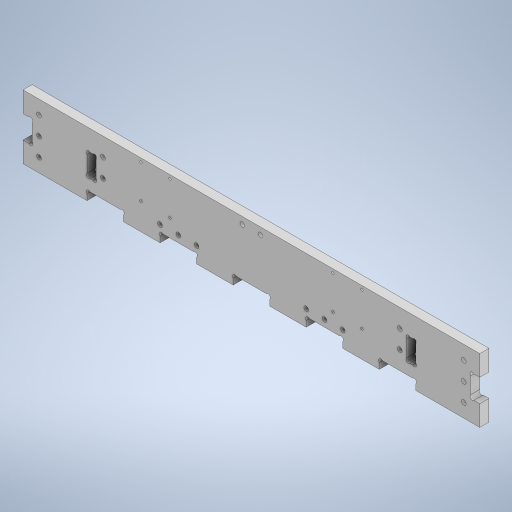
# Autodesk Inventor part: Back Wall
Saved by Autodesk Inventor 2023 (Build 270158000, 158)
## iProperties
Created: 2022-12-26
Part Number: Back Wall
Material: Generic
Document SubType Name: Modeling
Designer: justi
Density: 1 g/cm^3
Appearance: Default
Mass: 647.44 g
Surface Area: 1291.94 cm^2
Volume: 647.44 cm^3
Author: justi
Autodesk Inventor part; units mm, degrees
ref_plane "YZ Plane" through (0, 0, 0) normal (1, 0, 0) x (0, 1, 0)
ref_plane "XZ Plane" through (0, 0, 0) normal (0, 1, 0) x (-1, 0, 0)
ref_plane "XY Plane" through (0, 0, 0) normal (0, 0, 1) x (1, 0, 0)
sketch "Sketch1" plane through (0, 0, 0) normal (0, 0, 1) x (1, 0, 0)
  line L0 (0, 0) -> (457.2, 0)
  line L1 (457.2, 0) -> (457.2, 88.9)
  line L2 (457.2, 88.9) -> (0, 88.9)
  line L3 (0, 88.9) -> (0, 0)
  line L4 (0, 0) -> (50.8, 0)
  line L5 (50.8, 0) -> (50.8, 12.7)
  line L6 (50.8, 12.7) -> (0, 12.7)
  line L7 (0, 12.7) -> (0, 0)
  line L8 (457.2, 0) -> (406.4, 0)
  line L9 (406.4, 0) -> (406.4, 12.7)
  line L10 (406.4, 12.7) -> (457.2, 12.7)
  line L11 (457.2, 12.7) -> (457.2, 0)
  line L12 (101.6, 0) -> (152.4, 0)
  line L13 (152.4, 0) -> (152.4, 12.7)
  line L14 (152.4, 12.7) -> (101.6, 12.7)
  line L15 (101.6, 12.7) -> (101.6, 0)
  line L16 (355.6, 0) -> (304.8, 0)
  line L17 (304.8, 0) -> (304.8, 12.7)
  line L18 (304.8, 12.7) -> (355.6, 12.7)
  line L19 (355.6, 12.7) -> (355.6, 0)
  line L20 (254, 0) -> (203.2, 0)
  line L21 (203.2, 0) -> (203.2, 12.7)
  line L22 (203.2, 12.7) -> (254, 12.7)
  line L23 (254, 12.7) -> (254, 0)
  line L24 (0, 60.325) -> (12.7, 60.325)
  line L25 (12.7, 60.325) -> (12.7, 28.575)
  line L26 (12.7, 28.575) -> (0, 28.575)
  line L27 (0, 28.575) -> (0, 60.325)
  line L28 (457.2, 60.325) -> (444.5, 60.325)
  line L29 (444.5, 60.325) -> (444.5, 28.575)
  line L30 (444.5, 28.575) -> (457.2, 28.575)
  line L31 (457.2, 28.575) -> (457.2, 60.325)
  line L32 (0, 88.9) -> (-88.9, 88.9)
  line L33 (-88.9, 88.9) -> (-88.9, 0)
  line L34 (-88.9, 0) -> (0, 0)
  line L35 (0, 0) -> (0, 88.9)
  line L36 (-88.9, 60.325) -> (-76.2, 60.325)
  line L37 (-76.2, 60.325) -> (-76.2, 28.575)
  line L38 (-76.2, 28.575) -> (-88.9, 28.575)
  line L39 (-88.9, 28.575) -> (-88.9, 60.325)
  line L40 (457.2, 88.9) -> (546.1, 88.9)
  line L41 (546.1, 88.9) -> (546.1, 0)
  line L42 (546.1, 0) -> (457.2, 0)
  line L43 (457.2, 0) -> (457.2, 88.9)
  line L44 (546.1, 60.325) -> (533.4, 60.325)
  line L45 (533.4, 60.325) -> (533.4, 28.575)
  line L46 (533.4, 28.575) -> (546.1, 28.575)
  line L47 (546.1, 28.575) -> (546.1, 60.325)
  point P0 (0, 28.575)
  dimension "d0" = 457.2
  dimension "d1" = 88.9
  dimension "d2" = 50.8
  dimension "d3" = 12.7
  dimension "d4" = 50.8
  dimension "d5" = 12.7
  dimension "d6" = 50.8
  dimension "d7" = 12.7
  dimension "d8" = 50.8
  dimension "d9" = 50.8
  dimension "d10" = 12.7
  dimension "d11" = 50.8
  dimension "d12" = 50.8
  dimension "d13" = 12.7
  dimension "d14" = 50.8
  dimension "d15" = 12.7
  dimension "d16" = 15.875
  dimension "d17" = 28.575
  dimension "d18" = 12.7
  dimension "d19" = 28.575
  dimension "d20" = 15.875
  dimension "d21" = 88.9
  dimension "d22" = 12.7
  dimension "d23" = 28.575
  dimension "d24" = 31.75
  dimension "d25" = 88.9
  dimension "d26" = 12.7
  dimension "d27" = 28.575
  dimension "d28" = 31.75
  constraints: 96 end point, 24 parallel, 12 horizontal, 12 perpendicular, 7 point on line
  measures "d0" distance of L1.end L2.end
  measures "d1" distance of L0.end L1.end
  measures "d2" distance of L6.end L5.end
  measures "d3" distance of L4.end L5.end
  measures "d4" distance of L9.end L10.end
  measures "d5" distance of L8.end L9.end
  measures "d6" distance of L14.end L13.end
  measures "d7" distance of L12.end L13.end
  measures "d8" distance between parallel lines of L5 L15
  measures "d9" distance of L17.end L18.end
  measures "d10" distance of L16.end L17.end
  measures "d11" distance between parallel lines of L9 L19
  measures "d12" distance of L21.end L22.end
  measures "d13" distance of L20.end L21.end
  measures "d14" distance between parallel lines of L17 L23
  measures "d15" distance of L25.end L26.end
  measures "d16" distance between parallel lines of L6 L26
  measures "d17" distance between parallel lines of L2 L24
  measures "d18" distance of L30.end L29.end
  measures "d19" distance between parallel lines of L2 L28
  measures "d20" distance between parallel lines of L10 L30
  measures "d21" distance of L34.end L33.end
  measures "d22" distance of L37.end L38.end
  measures "d23" distance between parallel lines of L32 L36
  measures "d24" distance of L36.end L37.end
  measures "d25" distance of L41.end L42.end
  measures "d26" distance of L46.end L45.end
  measures "d27" distance between parallel lines of L40 L44
  measures "d28" distance of L44.end L45.end
extrude "Extrusion1" add sketch "Sketch1" along normal blind 12.7 contours L34 L33 L38 L37 L36 L32 L3 | L5 L6 L3 L26 L25 L24 L2 L1 L28 L29 L30 L10 L9 L0 L19 L18 L17 L23 L22 L21 L13 L14 L15 | L40 L41 L44 L45 L46 L42 L1
sketch "Sketch2" plane through (0, 0, 12.7) normal (0, 0, 1) x (1, 0, 0)
  line L0 (-76.2, 60.325) -> (-76.2, 28.575) projected
  line L1 (-76.2, 60.325) -> (-78.4451, 58.0799)
  line L2 (-76.2, 28.575) -> (-78.4451, 30.8201)
  line L3 (0, 28.575) -> (0, 60.325) projected
  line L4 (0, 60.325) -> (2.2451, 58.0799)
  line L5 (0, 60.325) -> (12.7, 60.325) projected
  line L6 (12.7, 60.325) -> (10.4549, 58.0799)
  line L7 (12.7, 60.325) -> (12.7, 28.575) projected
  line L8 (12.7, 28.575) -> (0, 28.575) projected
  line L9 (0, 28.575) -> (2.2451, 30.8201)
  line L10 (12.7, 60.325) -> (12.7, 28.575) projected
  line L11 (12.7, 28.575) -> (10.4549, 30.8201)
  line L12 (0, 0) -> (0, 12.7) projected
  line L13 (0, 12.7) -> (2.2451, 10.4549)
  line L14 (0, 12.7) -> (50.8, 12.7) projected
  line L15 (50.8, 12.7) -> (50.8, 0) projected
  line L16 (50.8, 12.7) -> (48.5549, 10.4549)
  line L17 (101.6, 0) -> (101.6, 12.7) projected
  line L18 (101.6, 12.7) -> (103.8451, 10.4549)
  line L19 (101.6, 12.7) -> (152.4, 12.7) projected
  line L20 (152.4, 12.7) -> (152.4, 0) projected
  line L21 (152.4, 12.7) -> (150.1549, 10.4549)
  line L22 (203.2, 0) -> (203.2, 12.7) projected
  line L23 (203.2, 12.7) -> (205.4451, 10.4549)
  line L24 (203.2, 12.7) -> (254, 12.7) projected
  line L25 (254, 12.7) -> (254, 0) projected
  line L26 (254, 12.7) -> (251.7549, 10.4549)
  line L27 (304.8, 0) -> (304.8, 12.7) projected
  line L28 (304.8, 12.7) -> (307.0451, 10.4549)
  line L29 (304.8, 12.7) -> (355.6, 12.7) projected
  line L30 (355.6, 12.7) -> (355.6, 0) projected
  line L31 (355.6, 12.7) -> (353.3549, 10.4549)
  line L32 (406.4, 0) -> (406.4, 12.7) projected
  line L33 (406.4, 12.7) -> (408.6451, 10.4549)
  line L34 (406.4, 12.7) -> (457.2, 12.7) projected
  line L35 (457.2, 12.7) -> (454.9549, 10.4549)
  line L36 (457.2, 12.7) -> (457.2, 0) projected
  line L37 (444.5, 28.575) -> (444.5, 60.325) projected
  line L38 (444.5, 60.325) -> (446.7451, 58.0799)
  line L39 (444.5, 60.325) -> (457.2, 60.325) projected
  line L40 (457.2, 60.325) -> (457.2, 28.575) projected
  line L41 (457.2, 60.325) -> (454.9549, 58.0799)
  line L42 (444.5, 28.575) -> (446.7451, 30.8201)
  line L43 (457.2, 28.575) -> (444.5, 28.575) projected
  line L44 (457.2, 28.575) -> (454.9549, 30.8201)
  line L45 (533.4, 28.575) -> (533.4, 60.325) projected
  line L46 (533.4, 60.325) -> (535.6451, 58.0799)
  line L47 (533.4, 60.325) -> (546.1, 60.325) projected
  line L48 (546.1, 28.575) -> (533.4, 28.575) projected
  line L49 (533.4, 28.575) -> (535.6451, 30.8201)
  circle A0 centre (-78.4451, 58.0799) radius 3.175
  circle A1 centre (-78.4451, 30.8201) radius 3.175
  circle A2 centre (2.2451, 58.0799) radius 3.175
  circle A3 centre (10.4549, 58.0799) radius 3.175
  circle A4 centre (2.2451, 30.8201) radius 3.175
  circle A5 centre (10.4549, 30.8201) radius 3.175
  circle A6 centre (2.2451, 10.4549) radius 3.175
  circle A7 centre (48.5549, 10.4549) radius 3.175
  circle A8 centre (103.8451, 10.4549) radius 3.175
  circle A9 centre (150.1549, 10.4549) radius 3.175
  circle A10 centre (205.4451, 10.4549) radius 3.175
  circle A11 centre (251.7549, 10.4549) radius 3.175
  circle A12 centre (307.0451, 10.4549) radius 3.175
  circle A13 centre (353.3549, 10.4549) radius 3.175
  circle A14 centre (408.6451, 10.4549) radius 3.175
  circle A15 centre (454.9549, 10.4549) radius 3.175
  circle A16 centre (446.7451, 30.8201) radius 3.175
  circle A17 centre (454.9549, 30.8201) radius 3.175
  circle A18 centre (454.9549, 58.0799) radius 3.175
  circle A19 centre (446.7451, 58.0799) radius 3.175
  circle A20 centre (535.6451, 58.0799) radius 3.175
  circle A21 centre (535.6451, 30.8201) radius 3.175
  dimension "d31" = 3.175
  dimension "d32" = 45
  dimension "d33" = 3.175
  dimension "d34" = 45
  dimension "d35" = 3.175
  dimension "d36" = 45
  dimension "d37" = 3.175
  dimension "d38" = 45
  dimension "d39" = 3.175
  dimension "d40" = 45
  dimension "d41" = 3.175
  dimension "d42" = 45
  dimension "d43" = 3.175
  dimension "d44" = 45
  dimension "d45" = 3.175
  dimension "d46" = 45
  dimension "d47" = 3.175
  dimension "d48" = 45
  dimension "d49" = 3.175
  dimension "d50" = 45
  dimension "d51" = 3.175
  dimension "d52" = 45
  dimension "d53" = 3.175
  dimension "d54" = 45
  dimension "d55" = 3.175
  dimension "d56" = 45
  dimension "d57" = 3.175
  dimension "d58" = 45
  dimension "d59" = 3.175
  dimension "d60" = 45
  dimension "d61" = 3.175
  dimension "d62" = 45
  dimension "d63" = 3.175
  dimension "d64" = 45
  dimension "d65" = 3.175
  dimension "d66" = 45
  dimension "d67" = 3.175
  dimension "d68" = 45
  dimension "d69" = 3.175
  dimension "d70" = 45
  dimension "d71" = 3.175
  dimension "d72" = 45
  dimension "d73" = 3.175
  dimension "d74" = 45
  dimension "d75" = 6.35
  dimension "d76" = 6.35
  dimension "d77" = 6.35
  dimension "d78" = 6.35
  dimension "d79" = 6.35
  dimension "d80" = 6.35
  dimension "d81" = 6.35
  dimension "d82" = 6.35
  dimension "d83" = 6.35
  dimension "d84" = 6.35
  dimension "d85" = 6.35
  dimension "d86" = 6.35
  dimension "d87" = 6.35
  dimension "d88" = 6.35
  dimension "d89" = 6.35
  dimension "d90" = 6.35
  dimension "d91" = 6.35
  dimension "d92" = 6.35
  dimension "d93" = 6.35
  dimension "d94" = 6.35
  constraints: 44 end point, 22 centre point, 14 point on line, 1 coincident
  measures "d31" distance of L0.start L1.end
  measures "d32" angle of L0 L1
  measures "d33" distance of L0.end L2.end
  measures "d34" angle of L0 L2
  measures "d35" distance of L3.end L4.end
  measures "d36" angle of L5 L4
  measures "d37" distance of L5.end L6.end
  measures "d38" angle of L7 L6
  measures "d39" distance of L3.start L9.end
  measures "d40" angle of L8 L9
  measures "d41" distance of L7.end L11.end
  measures "d42" angle of L7 L11
  measures "d43" distance of L12.end L13.end
  measures "d44" angle of L14 L13
  measures "d45" distance of L14.end L16.end
  measures "d46" angle of L15 L16
  measures "d47" distance of L17.end L18.end
  measures "d48" angle of L19 L18
  measures "d49" distance of L19.end L21.end
  measures "d50" angle of L20 L21
  measures "d51" distance of L22.end L23.end
  measures "d52" angle of L24 L23
  measures "d53" distance of L24.end L26.end
  measures "d54" angle of L25 L26
  measures "d55" distance of L27.end L28.end
  measures "d56" angle of L29 L28
  measures "d57" distance of L29.end L31.end
  measures "d58" angle of L30 L31
  measures "d59" distance of L32.end L33.end
  measures "d60" angle of L34 L33
  measures "d61" distance of L34.end L35.end
  measures "d62" angle of L36 L35
  measures "d63" distance of L37.end L38.end
  measures "d64" angle of L39 L38
  measures "d65" distance of L39.end L41.end
  measures "d66" angle of L40 L41
  measures "d67" distance of L37.start L42.end
  measures "d68" angle of L43 L42
  measures "d69" distance of L40.end L44.end
  measures "d70" angle of L40 L44
  measures "d71" distance of L45.end L46.end
  measures "d72" angle of L47 L46
  measures "d73" distance of L45.start L49.end
  measures "d74" angle of L48 L49
  measures "d75" diameter of A0
  measures "d76" diameter of A1
  measures "d77" diameter of A2
  measures "d78" diameter of A3
  measures "d79" diameter of A4
  measures "d80" diameter of A5
  measures "d81" diameter of A6
  measures "d82" diameter of A7
  measures "d83" diameter of A8
  measures "d84" diameter of A9
  measures "d85" diameter of A10
  measures "d86" diameter of A11
  measures "d87" diameter of A12
  measures "d88" diameter of A13
  measures "d89" diameter of A14
  measures "d90" diameter of A15
  measures "d91" diameter of A16
  measures "d92" diameter of A17
  measures "d93" diameter of A18
  measures "d94" diameter of A19
extrude "Extrusion2" cut sketch "Sketch2" against normal blind 12.7 contours A0 L0 | A1 L0 | L0 A1 | L0 A0 | A4 L3 | L3 A4 L8 | L8 A4 | A2 L3 | L3 L5 A2 | A5 L7 L8 | L8 A5 | A2 L5 | L7 A5 | A3 L5 L7 | L7 A3 | A3 L5 | A6 L12 | A7 L14 | L14 L15 A7 | L12 L14 A6 | A6 L14 | A7 L15 | A8 L17 | A9 L19 | L19 L20 A9 | L17 L19 A8 | A8 L19 | A9 L20 | A10 L22 | A11 L24 | L24 L25 A11 | L22 L24 A10 | A10 L24 | A11 L25 | A12 L27 | A13 L29 | L29 L30 A13 | L27 L29 A12 | A12 L29 | A13 L30 | A14 L32 | A15 L34 | L34 L36 A15 | L32 L34 A14 | A14 L34 | A15 L36 | A16 L37 | L37 A16 L43 | L43 A16 | A19 L37 | L37 L39 A19 | A17 L40 L43 | L43 A17 | A19 L39 | L40 A17 | A18 L39 L40 | L40 A18 | A18 L39 | A21 L45 | L45 A21 L48 | A20 L45 | L45 L47 A20 | L48 A21 | A20 L47
sketch "Sketch3" plane through (0, 0, 12.7) normal (0, 0, 1) x (1, 0, 0)
  circle A0 centre (127, 22.225) radius 3.175
  line L0 (106.0901, 12.7) -> (147.9099, 12.7) projected
  line L1 (101.6, 0) -> (101.6, 8.2099) projected
  circle A1 centre (101.6, 22.225) radius 3.175
  circle A2 centre (152.4, 22.225) radius 3.175
  circle A3 centre (330.2, 22.225) radius 3.175
  line L2 (309.2901, 12.7) -> (351.1099, 12.7) projected
  line L3 (355.6, 8.2099) -> (355.6, 0) projected
  circle A4 centre (304.8, 22.225) radius 3.175
  circle A5 centre (355.6, 22.225) radius 3.175
  circle A6 centre (22.225, 38.1) radius 3.175
  line L4 (4.4901, 12.7) -> (46.3099, 12.7) projected
  line L5 (12.7, 55.8349) -> (12.7, 33.0651) projected
  circle A7 centre (22.225, 63.5) radius 3.175
  circle A8 centre (434.975, 38.1) radius 3.175
  line L6 (444.5, 33.0651) -> (444.5, 55.8349) projected
  line L7 (410.8901, 12.7) -> (452.7099, 12.7) projected
  circle A9 centre (434.975, 63.5) radius 3.175
  circle A10 centre (-66.675, 44.45) radius 3.175
  line L8 (546.1, 88.9) -> (-88.9, 88.9) projected
  line L9 (-76.2, 55.8349) -> (-76.2, 33.0651) projected
  circle A11 centre (-66.675, 69.85) radius 3.175
  circle A12 centre (-66.675, 19.05) radius 3.175
  circle A13 centre (523.875, 44.45) radius 3.175
  line L10 (533.4, 33.0651) -> (533.4, 55.8349) projected
  circle A14 centre (523.875, 69.85) radius 3.175
  circle A15 centre (523.875, 19.05) radius 3.175
  point P0 (0, 0)
  dimension "d99" = 6.35
  dimension "d100" = 9.525
  dimension "d101" = 25.4
  dimension "d102" = 6.35
  dimension "d103" = 9.525
  dimension "d104" = 25.4
  dimension "d105" = 6.35
  dimension "d106" = 25.4
  dimension "d107" = 9.525
  dimension "d108" = 6.35
  dimension "d109" = 9.525
  dimension "d110" = 25.4
  dimension "d111" = 6.35
  dimension "d112" = 9.525
  dimension "d113" = 25.4
  dimension "d114" = 6.35
  dimension "d115" = 25.4
  dimension "d116" = 9.525
  dimension "d117" = 6.35
  dimension "d118" = 25.4
  dimension "d119" = 9.525
  dimension "d120" = 6.35
  dimension "d121" = 9.525
  dimension "d122" = 25.4
  dimension "d123" = 6.35
  dimension "d124" = 9.525
  dimension "d125" = 25.4
  dimension "d126" = 6.35
  dimension "d127" = 9.525
  dimension "d128" = 25.4
  dimension "d129" = 6.35
  dimension "d130" = 44.45
  dimension "d131" = 9.525
  dimension "d132" = 6.35
  dimension "d133" = 9.525
  dimension "d134" = 25.4
  dimension "d135" = 6.35
  dimension "d136" = 9.525
  dimension "d137" = 25.4
  dimension "d138" = 6.35
  dimension "d139" = 9.525
  dimension "d140" = 44.45
  dimension "d141" = 6.35
  dimension "d142" = 9.525
  dimension "d143" = 25.4
  dimension "d144" = 6.35
  dimension "d145" = 9.525
  dimension "d146" = 25.4
  constraints: 16 centre point
  measures "d99" diameter of A0
  measures "d100" distance from line of L0 A0.centre
  measures "d101" distance from line of L1 A0.centre
  measures "d102" diameter of A1
  measures "d103" distance from line of L0 A1.centre
  measures "d104" distance of A0.centre A1.centre
  measures "d105" diameter of A2
  measures "d106" distance of A0.centre A2.centre
  measures "d107" distance from line of L0 A2.centre
  measures "d108" diameter of A3
  measures "d109" distance from line of L2 A3.centre
  measures "d110" distance from line of L3 A3.centre
  measures "d111" diameter of A4
  measures "d112" distance from line of L2 A4.centre
  measures "d113" distance of A3.centre A4.centre
  measures "d114" diameter of A5
  measures "d115" distance of A3.centre A5.centre
  measures "d116" distance from line of L2 A5.centre
  measures "d117" diameter of A6
  measures "d118" distance from line of L4 A6.centre
  measures "d119" distance from line of L5 A6.centre
  measures "d120" diameter of A7
  measures "d121" distance from line of L5 A7.centre
  measures "d122" distance of A6.centre A7.centre
  measures "d123" diameter of A8
  measures "d124" distance from line of L6 A8.centre
  measures "d125" distance from line of L7 A8.centre
  measures "d126" diameter of A9
  measures "d127" distance from line of L6 A9.centre
  measures "d128" distance of A8.centre A9.centre
  measures "d129" diameter of A10
  measures "d130" distance from line of L8 A10.centre
  measures "d131" distance from line of L9 A10.centre
  measures "d132" diameter of A11
  measures "d133" distance from line of L9 A11.centre
  measures "d134" distance of A10.centre A11.centre
  measures "d135" diameter of A12
  measures "d136" distance from line of L9 A12.centre
  measures "d137" distance of A10.centre A12.centre
  measures "d138" diameter of A13
  measures "d139" distance from line of L10 A13.centre
  measures "d140" distance from line of L8 A13.centre
  measures "d141" diameter of A14
  measures "d142" distance from line of L10 A14.centre
  measures "d143" distance of A13.centre A14.centre
  measures "d144" diameter of A15
  measures "d145" distance from line of L10 A15.centre
  measures "d146" distance of A13.centre A15.centre
extrude "Extrusion3" cut sketch "Sketch3" against normal blind 12.7
sketch "Sketch6" plane through (0, 0, 12.7) normal (0, 0, 1) x (1, 0, 0)
  circle A0 centre (115.2922, 36.9094) radius 1.5875
  circle A1 centre (127, 22.225) radius 3.175 projected
  circle A2 centre (115.2922, 83.7406) radius 1.5875
  line L0 (88.9, 31.75) -> (165.1, 31.75)
  line L1 (165.1, 31.75) -> (165.1, 12.7)
  line L2 (165.1, 12.7) -> (88.9, 12.7)
  line L3 (88.9, 12.7) -> (88.9, 31.75)
  line L4 (88.9, 31.75) -> (165.1, 12.7) construction
  line L5 (165.1, 31.75) -> (88.9, 12.7) construction
  line L6 (546.1, 88.9) -> (-88.9, 88.9) projected
  line L7 (292.1, 31.75) -> (368.3, 31.75)
  line L8 (368.3, 31.75) -> (368.3, 12.7)
  line L9 (368.3, 12.7) -> (292.1, 12.7)
  line L10 (292.1, 12.7) -> (292.1, 31.75)
  circle A3 centre (330.2, 22.225) radius 3.175 projected
  line L11 (292.1, 31.75) -> (368.3, 12.7) construction
  line L12 (368.3, 31.75) -> (292.1, 12.7) construction
  circle A4 centre (341.9078, 36.9094) radius 1.5875
  circle A5 centre (341.9078, 83.7406) radius 1.5875
  circle A6 centre (75.0094, 83.7406) radius 1.5875
  circle A7 centre (75.0094, 36.9094) radius 1.5875
  circle A8 centre (382.1906, 36.9094) radius 1.5875
  circle A9 centre (382.1906, 83.7406) radius 1.5875
  point P0 (0, 0)
  dimension "d149" = 3.175
  dimension "d150" = 11.7078
  dimension "d151" = 3.175
  dimension "d152" = 46.8312
  dimension "d153" = 76.2
  dimension "d154" = 5.1594
  dimension "d155" = 5.1594
  dimension "d156" = 76.2
  dimension "d157" = 3.175
  dimension "d158" = 3.175
  dimension "d159" = 5.1594
  dimension "d160" = 11.7078
  dimension "d161" = 46.8312
  dimension "d162" = 5.1594
  dimension "d163" = 3.175
  dimension "d164" = 3.175
  dimension "d165" = 5.1594
  dimension "d166" = 40.2828
  dimension "d167" = 40.2828
  dimension "d168" = 46.8312
  dimension "d169" = 3.175
  dimension "d170" = 5.1594
  dimension "d171" = 40.2828
  dimension "d172" = 3.175
  dimension "d173" = 46.8312
  dimension "d174" = 40.2828
  constraints: 24 end point, 8 centre point, 4 midpoint, 4 parallel, 2 horizontal, 2 perpendicular
  measures "d149" diameter of A0
  measures "d150" horizontal distance of A0.centre A1.centre
  measures "d151" diameter of A2
  measures "d152" distance of A0.centre A2.centre
  measures "d153" distance of L1.end L2.end
  measures "d154" distance from line of L6 A2.centre
  measures "d155" distance from line of L0 A0.centre
  measures "d156" distance of L8.end L9.end
  measures "d157" diameter of A4
  measures "d158" diameter of A5
  measures "d159" distance from line of L7 A4.centre
  measures "d160" horizontal distance of A3.centre A4.centre
  measures "d161" distance of A4.centre A5.centre
  measures "d162" distance from line of L6 A5.centre
  measures "d163" diameter of A6
  measures "d164" diameter of A7
  measures "d165" distance from line of L0 A7.centre
  measures "d166" distance of A0.centre A7.centre
  measures "d167" distance of A2.centre A6.centre
  measures "d168" distance of A7.centre A6.centre
  measures "d169" diameter of A8
  measures "d170" distance from line of L7 A8.centre
  measures "d171" distance of A4.centre A8.centre
  measures "d172" diameter of A9
  measures "d173" distance of A8.centre A9.centre
  measures "d174" distance of A5.centre A9.centre
extrude "Extrusion4" cut sketch "Sketch6" against normal blind 12.7 contours A0 | A2 | A4 | A5 | A6 | A7 | A8 | A9
sketch "Sketch8" plane through (0, 0, 12.7) normal (0, 0, 1) x (1, 0, 0)
  circle A0 centre (215.9, 79.375) radius 3.175
  circle A1 centre (241.3, 79.375) radius 3.175
  line L0 (546.1, 88.9) -> (-88.9, 88.9) projected
  line L1 (203.2, 0) -> (203.2, 8.2099) projected
  point P0 (0, 0)
  dimension "d188" = 6.35
  dimension "d189" = 6.35
  dimension "d190" = 9.525
  dimension "d191" = 9.525
  dimension "d192" = 25.4
  dimension "d193" = 12.7
  constraints: 2 centre point
  measures "d188" diameter of A0
  measures "d189" diameter of A1
  measures "d190" distance from line of L0 A0.centre
  measures "d191" distance from line of L0 A1.centre
  measures "d192" distance of A1.centre A0.centre
  measures "d193" distance from line of L1 A0.centre
extrude "Extrusion6" cut sketch "Sketch8" against normal blind 12.7
body "Solid1"
